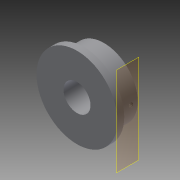
# Autodesk Inventor part: CapHolder
Saved by Autodesk Inventor 2015 SP2 (Build 190223200, 223)
## iProperties
Created: 2016-03-05
Part Number: CapHolder
Material: Generic
Document SubType Name: Modeling
Designer: marc
Density: 1 g/cm^3
Appearance: Default
Author: marc
Autodesk Inventor part; units mm, degrees
ref_plane "XZ Plane" through (0, 0, 0) normal (0, 1, 0) x (-1, 0, 0)
ref_plane "XY Plane" through (0, 0, 0) normal (0, 0, 1) x (1, 0, 0)
sketch "Sketch1" plane through (0, 0, 0) normal (0, 1, 0) x (-1, 0, 0)
  circle A0 centre (0, 0) radius 30
  dimension "SyringeHolderCapD" = 60
  constraints: 1 centre point, 1 coincident
  measures "SyringeHolderCapD" diameter of A0
extrude "Extrusion1" add sketch "Sketch1" along normal blind 20
sketch "Sketch2" plane through (0, 20, 0) normal (0, 1, 0) x (1, 0, 0)
  circle A0 centre (0, 0) radius 30
  circle A1 centre (0, 0) radius 30 projected
  circle A2 centre (0, 0) radius 25
  dimension "FlangeThickness" = 5
  constraints: 2 centre point, 2 coincident, 1 concentric
  measures "FlangeThickness" radial gap between concentric circles of A0 A2
extrude "Extrusion2" cut sketch "Sketch2" against normal blind 15
sketch "Sketch3" plane through (0, 20, 0) normal (0, 1, 0) x (1, 0, 0)
  circle A0 centre (0, 0) radius 10
  dimension "syringeHole" = 20
  constraints: 1 centre point, 1 coincident
  measures "syringeHole" diameter of A0
extrude "Extrusion3" cut sketch "Sketch3" against normal through all
ref_plane "Work Plane1" through (30, 0, 0) normal (1, 0, 0) x (0, 1, 0)
sketch "Sketch4" plane through (30, 0, 0) normal (1, 0, 0) x (0, 1, 0)
  line L0 (0, 0) -> (27.9945, 0) construction
  line L1 (0, 30) -> (0, -30) construction
  point P0 (15, 0)
  dimension "d10" = 15
  constraints: 2 end point, 1 horizontal, 1 point on line
  measures "d10" distance from line of L1 point (15, 0)
hole "Hole1" at (30, 15, 0) direction (-1, 0, 0) diameter 3.242 end through all thread size "M4x0.7" class "6H" standard "ISO Metric profile"
body "Solid1"
